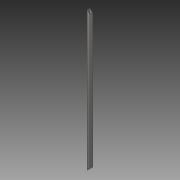
# Autodesk Inventor part: 1500mm_box_section
Saved by Autodesk Inventor 2019 (Build 230136000, 136)
## iProperties
Created: 2019-04-23
Part Number: 1500mm_box_section
Material: Steel, Mild
Document SubType Name: Modeling
Designer: Callum Snowden
Mass: 3173.36 g
Surface Area: 3241.78 cm^2
Volume: 404.25 cm^3
Density: 7.85 g/cm^3
Appearance: Semi-Polished
Author: Callum Snowden
Autodesk Inventor part; units mm, degrees
ref_plane "YZ Plane" through (0, 0, 0) normal (1, 0, 0) x (0, 1, 0)
ref_plane "XZ Plane" through (0, 0, 0) normal (0, 1, 0) x (-1, 0, 0)
ref_plane "XY Plane" through (0, 0, 0) normal (0, 0, 1) x (1, 0, 0)
sketch "Sketch1" plane through (0, 0, 0) normal (0, 1, 0) x (-1, 0, 0)
  line L0 (0, 0) -> (30, 0)
  line L1 (30, 0) -> (30, -30)
  line L2 (30, -30) -> (0, -30)
  line L3 (0, -30) -> (0, 0)
  line L4 (30, -15) -> (0, -15) construction
  line L5 (15, -30) -> (15, 0) construction
  line L6 (27.5, -2.5) -> (2.5, -2.5)
  line L7 (2.5, -2.5) -> (2.5, -27.5)
  line L8 (2.5, -27.5) -> (27.5, -27.5)
  line L9 (27.5, -27.5) -> (27.5, -2.5)
  dimension "d0" = 30
  dimension "d1" = 30
  dimension "d2" = 2.5
  dimension "d3" = 2.5
  constraints: 20 end point, 4 midpoint, 4 parallel, 2 horizontal, 2 perpendicular, 2 other
  measures "d0" distance of L1.end L2.end
  measures "d1" distance of L0.end L1.end
  measures "d2" distance between parallel lines of L6 L0
  measures "d3" distance between parallel lines of L1 L9
extrude "Extrusion1" add sketch "Sketch1" along normal blind 1500
sketch "Sketch2" plane through (0, 0, 0) normal (0, 0, 1) x (1, 0, 0)
  line L0 (0, 0) -> (-30, 0) construction
  line L1 (0, 0) -> (0, 1500) construction
  line L2 (-30, 1500) -> (0, 1500) construction
  line L3 (-30, 0) -> (-30, 1500) construction
  line L4 (0, 0) -> (-30, 0) projected
  line L5 (-30, 0) -> (0, 30)
  line L6 (-30, 0) -> (12.4264, 0) construction
  line L7 (-30, 1500) -> (0, 1470)
  line L8 (-30, 1500) -> (12.4264, 1500) construction
  dimension "d6" = 45
  dimension "d7" = 45
  constraints: 8 end point, 2 equal length, 2 horizontal, 2 point on line
  measures "d6" angle of L6 L5
  measures "d7" angle of L7 L8
extrude "Extrusion2" cut sketch "Sketch2" against normal up to surface (30 mm away) fills toward (-15.0354, 15.0354) keep common part open curves L5
extrude "Extrusion3" cut sketch "Sketch2" against normal up to surface (30 mm away) fills toward (-15.0354, 1484.9646) keep common part open curves L7
equation "\"d0\" = d1"
equation "\"d3\" = d2"
body "Solid1"
